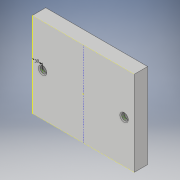
# Autodesk Inventor part: TablaInferior
Saved by Autodesk Inventor 2019 (Build 230136000, 136)
## iProperties
Created: 2019-05-15
Part Number: TablaInferior
Material: Generic
Document SubType Name: Modeling
Designer: Iván
Density: 1 g/cm^3
Appearance: Default
Author: Iván
Autodesk Inventor part; units mm, degrees
ref_plane "YZ Plane" through (0, 0, 0) normal (1, 0, 0) x (0, 1, 0)
ref_plane "XZ Plane" through (0, 0, 0) normal (0, 1, 0) x (-1, 0, 0)
ref_plane "XY Plane" through (0, 0, 0) normal (0, 0, 1) x (1, 0, 0)
sketch "Sketch1" plane through (0, 0, 0) normal (0, 0, 1) x (1, 0, 0)
  line L0 (-150, 125) -> (150, 125)
  line L1 (150, 125) -> (150, -125)
  line L2 (150, -125) -> (-150, -125)
  line L3 (-150, -125) -> (-150, 125)
  point P0 (0, 0)
  point P1 (0, 125)
  point P2 (150, 0)
  dimension "d0" = 300
  dimension "d1" = 250
  constraints: 8 end point, 2 midpoint, 2 parallel, 1 horizontal, 1 horizontal alignment, 1 perpendicular, 1 vertical alignment
  measures "d0" distance of L0.start L0.end
  measures "d1" distance of L0.end L1.end
extrude "Extrusion1" add sketch "Sketch1" along normal blind 39.37
sketch "Sketch2" plane through (0, 0, 39.37) normal (0, 0, 1) x (1, 0, 0)
  line L0 (-150, 125) -> (-150, -125) projected
  line L1 (150, 125) -> (-150, 125) construction
  line L2 (0, 125) -> (0, -125) construction
  line L3 (-150, -125) -> (150, -125) construction
  point P0 (0, 0)
  point P1 (-120, 0)
  point P2 (120, 0)
  dimension "d4" = 30
  constraints: 2 end point, 2 midpoint, 1 symmetric about line
  measures "d4" distance from line of L0 point (-120, 0)
hole "Hole1" at (-120, 0, 39.37) at (120, 0, 39.37) direction (0, 0, -1) diameter 10 end through all
hole "Hole2" at (-120, 0, 39.37) at (120, 0, 39.37) direction (0, 0, -1) diameter 20 depth 10 tip angle 118 countersink diameter 25 countersink angle 82
body "Solid1"
